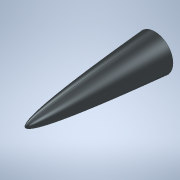
# Autodesk Inventor part: nose
Saved by Autodesk Inventor 2020 (Build 240168000, 168)
## iProperties
Created: 2021-01-23
Part Number: nose
Material: ABS Plastic
Document SubType Name: Modeling
Designer: 0x6f736f646f
Density: 1.06 g/cm^3
Appearance: Iron Gray
Author: 0x6f736f646f
Autodesk Inventor part; units mm, degrees
ref_plane "YZ Plane" through (0, 0, 0) normal (1, 0, 0) x (0, 1, 0)
ref_plane "XZ Plane" through (0, 0, 0) normal (0, 1, 0) x (-1, 0, 0)
ref_plane "XY Plane" through (0, 0, 0) normal (0, 0, 1) x (1, 0, 0)
sketch "Sketch1" plane through (0, 0, 0) normal (1, 0, 0) x (0, 1, 0)
  spline S0 degree 2 poles (16.8, 0) (7.4765, 120) (0, 120) knots 0 0 0 1 1 1
  spline S1 degree 2 poles (15, 0) (6.5777, 118.2) (0, 118.2) knots 0 0 0 1 1 1
  line L0 (-5.3333, 0) -> (24.382, 0) projected
  line L1 (0, 146.3795) -> (0, -25.9689) projected
  line L2 (16.8, 0) -> (15, 0)
  line L3 (0, 120) -> (0, 118.2)
  line L4 (0.9491, 118.2) -> (-0.9491, 118.2) construction
  arc A0 (0.527, 117.976) -> (-0.527, 117.976) centre (0, 117.4679) ccw construction
  line L5 (1.0883, 120) -> (-1.0883, 120) construction
  arc A1 (0.6361, 119.749) -> (-0.6361, 119.749) centre (0, 119.0684) ccw construction
  dimension "d55" = 1.8
  dimension "d57" = 120
  dimension "d58" = 118.2
  dimension "d59" = 16.8
  constraints: 8 end point, 4 midpoint, 3 horizontal, 2 centre point, 2 point on circle, 2 point on line, 1 vertical, 7 other
  measures "d55" distance of L2.end L2.start
  measures "d57" distance from line of L3.start L0
  measures "d58" distance from line of L3.end L0
  measures "d59" distance from line of L1 L2.start
revolve "Revolution4" add sketch "Sketch1" angle 360 about axis through (0, 0, 0) along (0, 0, -1) contours L0 S1 L1 S0
body "Solid3"
